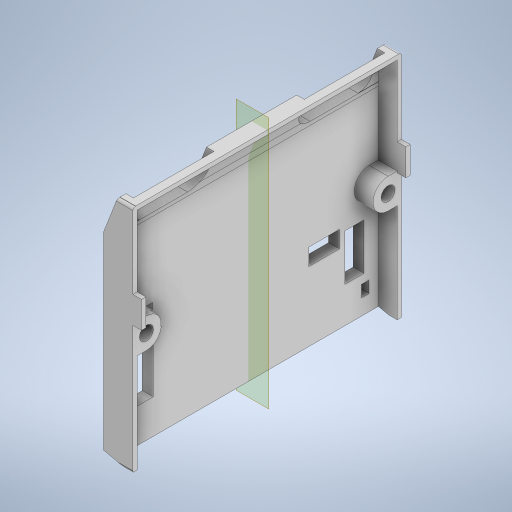
# Autodesk Inventor part: pokrywa
Saved by Autodesk Inventor 2023.5 (Build 275446000, 446)
## iProperties
Created: 2025-04-01
Part Number: pokrywa
Material: Ogólny
Document SubType Name: Modeling
Designer: kamil
Density: 1 g/cm^3
Appearance: Domyślna
Author: kamil
Autodesk Inventor part; units mm, degrees
ref_plane "YZ Plane" through (0, 0, 0) normal (1, 0, 0) x (0, 1, 0)
ref_plane "XZ Plane" through (0, 0, 0) normal (0, 1, 0) x (-1, 0, 0)
ref_plane "XY Plane" through (0, 0, 0) normal (0, 0, 1) x (1, 0, 0)
sketch "Szkic1" plane through (0, 0, 0) normal (1, 0, 0) x (0, 1, 0)
  line L0 (10.7442, -21.3655) -> (23.7442, -21.3655)
  line L1 (23.7442, -21.3655) -> (23.8098, -21.3634)
  arc A0 (23.8098, -21.3634) -> (24.2442, -20.8655) centre (23.7464, -20.8696) ccw
  line L2 (24.2442, -20.8655) -> (24.2442, 28.1345)
  line L3 (24.2442, 28.1345) -> (24.2421, 28.2)
  arc A1 (24.2421, 28.2) -> (23.7442, 28.6345) centre (23.7483, 28.1367) ccw
  line L4 (23.7442, 28.6345) -> (10.7442, 28.6345)
  line L5 (10.7442, 28.6345) -> (10.6787, 28.6324)
  line L6 (3.7484, 28.6345) -> (-18.1981, 28.6345)
  line L7 (-18.1981, 28.6345) -> (-18.2637, 28.6326)
  arc A2 (-18.2637, 28.6326) -> (-18.6981, 28.1345) centre (-18.2006, 28.139) ccw
  line L8 (-18.6981, 28.1345) -> (-18.6981, 27.1345)
  line L9 (-18.6981, 27.1345) -> (-18.6962, 27.0689)
  arc A3 (-18.6962, 27.0689) -> (-18.1981, 26.6345) centre (-18.2025, 27.1322) ccw
  line L10 (-18.1981, 26.6345) -> (-15.6162, 26.6345)
  line L11 (-15.6162, 26.6345) -> (-15.6162, 15.9345)
  line L12 (-15.6162, 15.9345) -> (-18.2023, 15.9345)
  line L13 (-18.2023, 15.9345) -> (-18.2679, 15.9326)
  arc A4 (-18.2679, 15.9326) -> (-18.7023, 15.4345) centre (-18.2048, 15.439) ccw
  line L14 (-18.7023, 15.4345) -> (-18.7023, -3.8655)
  line L15 (-18.7023, -3.8655) -> (-18.7004, -3.9311)
  arc A5 (-18.7004, -3.9311) -> (-18.2023, -4.3655) centre (-18.2067, -3.8678) ccw
  line L16 (-18.2023, -4.3655) -> (-15.6162, -4.3655)
  line L17 (-15.6162, -4.3655) -> (-15.6162, -15.0655)
  line L18 (-15.6162, -15.0655) -> (-18.2023, -15.0655)
  line L19 (-18.2023, -15.0655) -> (-18.2679, -15.0674)
  arc A6 (-18.2679, -15.0674) -> (-18.7023, -15.5655) centre (-18.2048, -15.561) ccw
  line L20 (-18.7023, -15.5655) -> (-18.7023, -20.8655)
  line L21 (-18.7023, -20.8655) -> (-18.7004, -20.9311)
  arc A7 (-18.7004, -20.9311) -> (-18.2023, -21.3655) centre (-18.2067, -20.8678) ccw
  line L22 (-18.2023, -21.3655) -> (3.7442, -21.3655)
  line L23 (3.7442, -21.3655) -> (3.8621, -21.3632)
  circle A8 centre (2.7442, 26.1345) radius 1.3
  circle A9 centre (2.7442, -18.8655) radius 1.3
  line L24 (10.7442, 28.6345) -> (3.7484, 28.6345)
  line L25 (3.7442, -21.3655) -> (10.7442, -21.3655)
  point P0 (0, 0)
  constraints: 52 end point, 16 point on circle, 10 centre point, 10 horizontal, 6 vertical, 1 parallel, 65 other
extrude "Wyciągnięcie proste1" add sketch "Szkic1" along normal blind 4
sketch "Szkic2" plane through (4, 0, 0) normal (1, 0, 0) x (0, 0, -1)
  line L0 (31.8312, -18.461) -> (-38.8363, -18.461)
  line L1 (21.3655, 23.7442) -> (21.3634, 23.8098) projected
  arc A0 (21.3634, 23.8098) -> (20.8655, 24.2442) centre (20.8696, 23.7464) ccw projected
  line L2 (20.8655, 24.2442) -> (-28.1345, 24.2442) projected
  line L3 (-28.1345, 24.2442) -> (-28.2, 24.2421) projected
  arc A1 (-28.2, 24.2421) -> (-28.6345, 23.7442) centre (-28.1367, 23.7483) ccw projected
  line L4 (-28.6345, 23.7442) -> (-28.6345, -18.1981) projected
  line L5 (-28.6345, -18.1981) -> (-28.6326, -18.2637) projected
  arc A2 (-28.6326, -18.2637) -> (-28.1345, -18.6981) centre (-28.139, -18.2006) ccw projected
  line L6 (-28.1345, -18.6981) -> (-27.1345, -18.6981) projected
  line L7 (-27.1345, -18.6981) -> (-27.0689, -18.6962) projected
  arc A3 (-27.0689, -18.6962) -> (-26.6345, -18.1981) centre (-27.1322, -18.2025) ccw projected
  line L8 (-26.6345, -18.1981) -> (-26.6345, -15.6162) projected
  line L9 (-26.6345, -15.6162) -> (-15.9345, -15.6162) projected
  line L10 (-15.9345, -15.6162) -> (-15.9345, -18.2023) projected
  line L11 (-15.9345, -18.2023) -> (-15.9326, -18.2679) projected
  arc A4 (-15.9326, -18.2679) -> (-15.4345, -18.7023) centre (-15.439, -18.2048) ccw projected
  line L12 (-15.4345, -18.7023) -> (3.8655, -18.7023) projected
  line L13 (3.8655, -18.7023) -> (3.9311, -18.7004) projected
  arc A5 (3.9311, -18.7004) -> (4.3655, -18.2023) centre (3.8678, -18.2067) ccw projected
  line L14 (4.3655, -18.2023) -> (4.3655, -15.6162) projected
  line L15 (4.3655, -15.6162) -> (15.0655, -15.6162) projected
  line L16 (15.0655, -15.6162) -> (15.0655, -18.2023) projected
  line L17 (15.0655, -18.2023) -> (15.0674, -18.2679) projected
  arc A6 (15.0674, -18.2679) -> (15.5655, -18.7023) centre (15.561, -18.2048) ccw projected
  line L18 (15.5655, -18.7023) -> (20.8655, -18.7023) projected
  line L19 (20.8655, -18.7023) -> (20.9311, -18.7004) projected
  arc A7 (20.9311, -18.7004) -> (21.3655, -18.2023) centre (20.8678, -18.2067) ccw projected
  line L20 (21.3655, -18.2023) -> (21.3655, 23.7442) projected
  circle A8 centre (-26.1345, 2.7442) radius 1.3 projected
  circle A9 centre (18.8655, 2.7442) radius 1.3 projected
  line L21 (20.8655, 24.2442) -> (-28.1345, 24.2442) projected
  point P0 (0, 0)
  point P1 (-26.7069, -18.461)
  point P2 (-15.8655, -18.461)
  point P3 (4.2957, -18.461)
  point P4 (15.1345, -18.461)
  point P5 (21.2957, -18.461)
  point P6 (-28.563, -18.461)
  constraints: 2 end point, 1 parallel
extrude "Wyciągnięcie proste2" add sketch "Szkic2" against normal up to surface (4 mm away) contours L0 A5 L14 L15 L16 L17 A6 | L0 A3 L8 L9 L10 L11 A4
extrude "Wyciągnięcie proste3" cut sketch "Szkic2" against normal through all contours A7 L19 L18 A6 L0 | A5 L13 L12 A4 L0 | A3 L7 L6 A2 L0
sketch "Szkic4" plane through (4, 0, 0) normal (1, 0, 0) x (0, 0, -1)
  circle A0 centre (18.8655, 2.7442) radius 1.3 projected
  circle A1 centre (-26.1345, 2.7442) radius 1.3 projected
  line L0 (-28.563, -18.461) -> (21.2957, -18.461) projected
  arc A2 (21.2957, -18.461) -> (21.3655, -18.2023) centre (20.8678, -18.2067) ccw projected
  line L1 (21.3655, -18.2023) -> (21.3655, 23.7442) projected
  line L2 (21.3655, 23.7442) -> (21.3634, 23.8098) projected
  arc A3 (21.3634, 23.8098) -> (20.8655, 24.2442) centre (20.8696, 23.7464) ccw projected
  line L3 (20.8655, 24.2442) -> (-28.1345, 24.2442) projected
  line L4 (-28.1345, 24.2442) -> (-28.2, 24.2421) projected
  arc A4 (-28.2, 24.2421) -> (-28.6345, 23.7442) centre (-28.1367, 23.7483) ccw projected
  line L5 (-28.6345, 23.7442) -> (-28.6345, -18.1981) projected
  line L6 (-28.6345, -18.1981) -> (-28.6326, -18.2637) projected
  arc A5 (-28.6326, -18.2637) -> (-28.563, -18.461) centre (-28.139, -18.2006) ccw projected
  line L7 (20.5655, 23.4442) -> (20.5655, -17.661)
  line L8 (20.5655, -17.661) -> (-27.8345, -17.661)
  line L9 (-27.8345, -17.661) -> (-27.8345, 23.4442)
  line L10 (-27.8345, 23.4442) -> (20.5655, 23.4442)
  circle A6 centre (18.8655, 2.7442) radius 2.8
  circle A7 centre (-26.1345, 2.7442) radius 2.8
  line L11 (18.8655, -0.0558) -> (20.5655, -0.0558)
  line L12 (20.5655, 5.5442) -> (18.8655, 5.5442)
  line L13 (-26.1345, -0.0558) -> (-27.8345, -0.0558)
  line L14 (-26.1345, 5.5442) -> (-27.8345, 5.5442)
  point P0 (0, 0)
  dimension "d8" = 0.8
  dimension "d9" = 1.5
  dimension "d10" = 1.5
  constraints: 16 end point, 4 perpendicular, 4 point on circle, 4 point on line, 4 tangent, 2 centre point, 3 other
  measures "d8" distance between parallel lines of L1 L7
  measures "d9" radial gap between concentric circles of A0 A6
  measures "d10" radial gap between concentric circles of A1 A7
extrude "Wyciągnięcie proste5" cut sketch "Szkic4" against normal blind 2 contours L7 L8 L9 L13 A7 L14 L10 L12 A6 L11
sketch "Szkic5" plane through (4, 0, 0) normal (1, 0, 0) x (0, 0, -1)
  line L0 (18.8655, -0.0558) -> (20.5655, -0.0558) projected
  line L1 (20.5655, -0.0558) -> (20.5655, -17.661) projected
  line L2 (20.5655, -17.661) -> (-27.8345, -17.661) projected
  line L3 (-27.8345, -17.661) -> (-27.8345, -0.0558) projected
  line L4 (-27.8345, -0.0558) -> (-26.1345, -0.0558) projected
  arc A0 (-26.1345, -0.0558) -> (-26.1345, 5.5442) centre (-26.1345, 2.7442) ccw projected
  line L5 (-26.1345, 5.5442) -> (-27.8345, 5.5442) projected
  line L6 (-27.8345, 5.5442) -> (-27.8345, 23.4442) projected
  line L7 (-27.8345, 23.4442) -> (20.5655, 23.4442) projected
  line L8 (20.5655, 23.4442) -> (20.5655, 5.5442) projected
  line L9 (20.5655, 5.5442) -> (18.8655, 5.5442) projected
  arc A1 (18.8655, 5.5442) -> (18.8655, -0.0558) centre (18.8655, 2.7442) ccw projected
  circle A2 centre (18.8655, 2.7442) radius 1.3 projected
  circle A3 centre (-26.1345, 2.7442) radius 1.3 projected
  line L10 (-28.563, -18.461) -> (21.2957, -18.461) projected
  arc A4 (21.2957, -18.461) -> (21.3655, -18.2023) centre (20.8678, -18.2067) ccw projected
  line L11 (21.3655, -18.2023) -> (21.3655, 23.7442) projected
  line L12 (21.3655, 23.7442) -> (21.3634, 23.8098) projected
  arc A5 (21.3634, 23.8098) -> (20.8655, 24.2442) centre (20.8696, 23.7464) ccw projected
  line L13 (20.8655, 24.2442) -> (-28.1345, 24.2442) projected
  line L14 (-28.1345, 24.2442) -> (-28.2, 24.2421) projected
  arc A6 (-28.2, 24.2421) -> (-28.6345, 23.7442) centre (-28.1367, 23.7483) ccw projected
  line L15 (-28.6345, 23.7442) -> (-28.6345, -18.1981) projected
  line L16 (-28.6345, -18.1981) -> (-28.6326, -18.2637) projected
  arc A7 (-28.6326, -18.2637) -> (-28.563, -18.461) centre (-28.139, -18.2006) ccw projected
  point P0 (0, 0)
extrude "Wyciągnięcie proste6" add sketch "Szkic5" along normal blind 1.5
sketch "Szkic9" plane through (0, 0, 0) normal (-1, 0, 0) x (0, 0, 1)
  line L0 (-21.2957, -18.461) -> (28.563, -18.461) projected
  arc A0 (28.563, -18.461) -> (28.6326, -18.2637) centre (28.139, -18.2006) ccw projected
  line L1 (28.6345, -18.1981) -> (28.6326, -18.2637) projected
  line L2 (28.6345, 23.7442) -> (28.6345, -18.1981) projected
  arc A1 (28.6345, 23.7442) -> (28.2, 24.2421) centre (28.1367, 23.7483) ccw projected
  line L3 (28.1345, 24.2442) -> (28.2, 24.2421) projected
  line L4 (-20.8655, 24.2442) -> (28.1345, 24.2442) projected
  arc A2 (-20.8655, 24.2442) -> (-21.3634, 23.8098) centre (-20.8696, 23.7464) ccw projected
  line L5 (-21.3655, 23.7442) -> (-21.3634, 23.8098) projected
  line L6 (-21.3655, -18.2023) -> (-21.3655, 23.7442) projected
  arc A3 (-21.3655, -18.2023) -> (-21.2957, -18.461) centre (-20.8678, -18.2067) ccw projected
  circle A4 centre (26.1345, 2.7442) radius 1.3 projected
  circle A5 centre (-18.8655, 2.7442) radius 1.3 projected
  line L7 (27.0345, 24.2442) -> (12.0345, 24.2442)
  line L8 (12.0345, 24.2442) -> (12.0345, 18.2442)
  line L9 (12.0345, 18.2442) -> (27.0345, 18.2442)
  line L10 (27.0345, 18.2442) -> (27.0345, 24.2442)
  line L11 (-19.7655, 24.2442) -> (-4.7655, 24.2442)
  line L12 (-4.7655, 24.2442) -> (-4.7655, 18.2442)
  line L13 (-4.7655, 18.2442) -> (-19.7655, 18.2442)
  line L14 (-19.7655, 18.2442) -> (-19.7655, 24.2442)
  line L15 (-20.8655, 24.2442) -> (28.1345, 24.2442) projected
  point P0 (0, 0)
  point P1 (-4.7655, 24.2442)
  point P2 (-19.7655, 24.2442)
  dimension "d20" = 15
  dimension "d21" = 15
  dimension "d22" = 1.6
  dimension "d23" = 1.6
  dimension "d24" = 6
  constraints: 16 end point, 4 parallel, 2 collinear, 2 horizontal, 2 perpendicular, 1 point on line
  measures "d20" distance between parallel lines of L8 L10
  measures "d21" distance between parallel lines of L14 L12
  measures "d22" distance between parallel lines of L10 L2
  measures "d23" distance between parallel lines of L6 L14
  measures "d24" distance between parallel lines of L7 L9
extrude "Wyciągnięcie proste9" cut sketch "Szkic9" against normal blind 4 contours L4 L12 L13 L14 | L10 L9 L8 L4
sketch "Szkic10" plane through (0, 18.2442, 12.0345) normal (0, 0, 1) x (1, 0, 0)
  line L0 (2, 5.2) -> (2, 0) projected
  line L1 (4, 5.2) -> (2, 5.2) projected
  line L2 (4, 5.2) -> (4, 6) projected
  line L3 (0, 6) -> (4, 6) projected
  line L4 (0, 0) -> (0, 6) projected
  line L5 (0, 0) -> (2, 0) projected
  line L6 (2, 5.2) -> (2, 0) projected
  line L7 (4, 5.2) -> (2, 5.2) projected
  line L8 (2, 0) -> (4, 5.2)
  point P0 (0, -18.2442)
  constraints: 2 end point
extrude "Wyciągnięcie proste10" add sketch "Szkic10" against normal up to surface (16.8 mm away) contours L1 L8 L0
sketch "Szkic11" plane through (0, -18.1981, 28.6345) normal (0, 0, 1) x (1, 0, 0)
  line L0 (2, 36.4423) -> (4, 41.6423) projected
  line L1 (-3.0884, 27.6697) -> (6.2618, 51.9802)
  line L2 (0, 42.4402) -> (0, 41.9423) projected
  line L3 (0, 41.9423) -> (5.5, 41.9423) projected
  line L4 (5.5, 42.4402) -> (5.5, 41.9423) projected
  line L5 (0, 42.4402) -> (5.5, 42.4402) projected
  line L6 (0, 41.9423) -> (0, 0) projected
  line L7 (0, 0) -> (5.5, 0) projected
  line L8 (5.5, 41.9423) -> (5.5, 0) projected
  line L9 (0, 41.9423) -> (5.5, 41.9423) projected
  line L10 (-3.0884, 27.6697) -> (-8.821, 53.9859)
  line L11 (-8.821, 53.9859) -> (6.2618, 51.9802)
  point P0 (0, 18.1981)
  dimension "d29" = 1.6
  constraints: 6 end point, 1 parallel
  measures "d29" distance between parallel lines of L1 L0
extrude "Wyciągnięcie proste11" cut sketch "Szkic11" along normal blind 10 and the other way blind 100 contours L10 L11 L1 L5 L2 L6 | L6 L3 L1 | L3 L2 L5 L1
sketch "Szkic12" plane through (2, 5.5442, -20.5655) normal (0, 0, 1) x (1, 0, 0)
  line L0 (0, 17.1571) -> (-1.7143, 12.7) projected
  line L1 (0.5934, 18.7) -> (0.2857, 17.9) projected
  line L2 (0.2857, 17.9) -> (0, 17.1571) projected
  line L3 (-0.7809, 12.341) -> (0.9333, 16.7981)
  line L4 (0.9333, 16.7981) -> (1.2191, 17.541)
  line L5 (1.2191, 17.541) -> (1.5268, 18.341)
  line L6 (0.2857, 17.9) -> (0, 17.1571) projected
  line L7 (0, 17.1571) -> (0, 0) projected
  line L8 (3.5, 0) -> (0, 0) projected
  line L9 (3.5, 17.9) -> (3.5, 0) projected
  line L10 (3.5, 17.9) -> (0.2857, 17.9) projected
  point P0 (-2, -5.5442)
  point P1 (1.3572, 17.9)
  point P2 (0, 14.3714)
  dimension "d34" = 1
  constraints: 6 end point, 2 other
  measures "d34" distance between parallel lines of L2 L4
extrude "Wyciągnięcie proste12" add sketch "Szkic12" along normal up to surface (0.8 mm away) contours L10 L5 L4 L3 L7 L2
ref_plane "Płaszczyzna konstrukcyjna1" through (5.5, -18.2023, 3.6345) normal (0, 0, -1) x (-1, 0, 0)
mirror "Odbij1" about plane through (5.5, -18.2023, 3.6345) normal (0, 0, -1) of "Wyciągnięcie proste12"
sketch "Szkic13" plane through (0, -18.1981, 28.6345) normal (0, 0, 1) x (1, 0, 0)
  line L0 (9.4474, -1.511) -> (-6.0785, 1.9749)
  line L1 (5.5, -0.2629) -> (0, -0.2629) projected
  line L2 (0, -0.2629) -> (0.1866, 0.5682)
  line L3 (0, -0.2629) -> (5.5, -0.2629) projected
  line L4 (5.5, -0.0656) -> (5.5, -0.2629) projected
  line L5 (0, -0.0656) -> (5.5, -0.0656) projected
  line L6 (0, -0.0656) -> (0, -0.2629) projected
  line L7 (2.4011, 41.9423) -> (0, 35.6994) projected
  line L8 (0, 35.6994) -> (0, 0) projected
  line L9 (0, 0) -> (5.5, 0) projected
  line L10 (5.5, 41.9423) -> (5.5, 0) projected
  line L11 (2.4011, 41.9423) -> (5.5, 41.9423) projected
  line L12 (0, 0) -> (5.5, 0) projected
  line L13 (0, 0) -> (0, -0.0656) projected
  line L14 (0, -0.0656) -> (5.5, -0.0656) projected
  line L15 (5.5, 0) -> (5.5, -0.0656) projected
  line L16 (0, 0) -> (5.5, 0) projected
  point P0 (0, 18.1981)
  point P1 (0, 0.6101)
  point P2 (3.8884, -0.2629)
  constraints: 4 end point, 1 perpendicular, 1 point on line
extrude "Wyciągnięcie proste13" cut sketch "Szkic13" against normal through all contours L1 L2 L5 L0 | L5 L2 L9 L0 | L6 L5 L2 | L9 L2 L0 | L5 L13 L9 L2 | L2 L9 L8 L0
sketch "Szkic14" plane through (0, 0, 0) normal (-1, 0, 0) x (0, 0, 1)
  line L0 (-15.0995, -3.2358) -> (-17.1315, -3.2358) projected
  line L1 (-17.1315, -10.8558) -> (-15.0995, -10.8558) projected
  line L2 (-17.3855, -8.5698) -> (-17.3855, -10.6018) projected
  line L3 (-14.8455, -5.5218) -> (-14.8455, -3.4898) projected
  line L4 (24.4295, -11.1458) -> (21.8895, -11.1458)
  line L5 (21.8895, -11.1458) -> (21.8895, -0.9858)
  line L6 (21.8895, -0.9858) -> (24.4295, -0.9858)
  line L7 (24.4295, -0.9858) -> (24.4295, -11.1458)
  line L8 (-17.3855, -10.8558) -> (-14.8455, -10.8558)
  line L9 (-14.8455, -10.8558) -> (-14.8455, -3.2358)
  line L10 (-14.8455, -3.2358) -> (-17.3855, -3.2358)
  line L11 (-17.3855, -3.2358) -> (-17.3855, -10.8558)
  line L12 (-14.3455, -2.7358) -> (-14.3455, -11.3558)
  line L13 (-14.3455, -11.3558) -> (-17.8855, -11.3558)
  line L14 (-17.8855, -11.3558) -> (-17.8855, -2.7358)
  line L15 (-17.8855, -2.7358) -> (-14.3455, -2.7358)
  line L16 (21.3895, -0.4858) -> (21.3895, -11.6458)
  line L17 (21.3895, -11.6458) -> (24.9295, -11.6458)
  line L18 (24.9295, -11.6458) -> (24.9295, -0.4858)
  line L19 (24.9295, -0.4858) -> (21.3895, -0.4858)
  point P0 (0, 0)
  dimension "d40" = 0.5
  dimension "d41" = 0.5
  constraints: 32 end point, 8 parallel, 4 perpendicular, 2 horizontal, 8 other
  measures "d40" distance between parallel lines of L9 L12
  measures "d41" distance between parallel lines of L5 L16
extrude "Wyciągnięcie proste14" cut sketch "Szkic14" against normal through all contours L10 L9 L3 L8 L1 L11 L2 L0 | L4 L5 L6 L7 | L12 L13 L14 L15 | L19 L18 L17 L16
sketch "Szkic15" plane through (0, 0, 0) normal (-1, 0, 0) x (0, 0, 1)
  line L0 (23.2345, 2.6442) -> (21.6645, 2.6442)
  line L1 (21.6645, 2.6442) -> (21.6645, 3.4442)
  line L2 (21.6645, 3.4442) -> (23.2345, 3.4442)
  line L3 (23.2345, 3.4442) -> (23.2345, 2.6442)
  line L4 (23.4345, 3.6442) -> (21.4645, 3.6442)
  line L5 (21.4645, 3.6442) -> (21.4645, 2.4442)
  line L6 (21.4645, 2.4442) -> (23.4345, 2.4442)
  line L7 (23.4345, 2.4442) -> (23.4345, 3.6442)
  point P0 (0, 0)
  dimension "d44" = 0.2
  constraints: 16 end point, 4 parallel, 2 perpendicular, 1 horizontal, 5 other
  measures "d44" distance between parallel lines of L2 L4
extrude "Wyciągnięcie proste15" cut sketch "Szkic15" against normal through all contours L0 L1 L2 L3 | L7 L6 L5 L4
sketch "Szkic16" plane through (0, 0, 0) normal (-1, 0, 0) x (0, 0, 1)
  line L0 (-18.5155, -13.2058) -> (-17.7155, -13.2058)
  line L1 (-17.7155, -13.2058) -> (-17.7155, -14.7758)
  line L2 (-17.7155, -14.7758) -> (-18.5155, -14.7758)
  line L3 (-18.5155, -14.7758) -> (-18.5155, -13.2058)
  line L4 (-17.4155, -15.0758) -> (-17.4155, -12.9058)
  line L5 (-17.4155, -12.9058) -> (-18.8155, -12.9058)
  line L6 (-18.8155, -12.9058) -> (-18.8155, -15.0758)
  line L7 (-18.8155, -15.0758) -> (-17.4155, -15.0758)
  point P0 (0, 0)
  dimension "d47" = 0.3
  constraints: 16 end point, 4 parallel, 2 perpendicular, 1 horizontal, 5 other
  measures "d47" distance between parallel lines of L1 L4
extrude "Wyciągnięcie proste16" cut sketch "Szkic16" against normal through all contours L0 L1 L2 L3 | L7 L6 L5 L4
sketch "Szkic17" plane through (5.5, 0, 0) normal (1, 0, 0) x (0, 0, -1)
  circle A0 centre (-26.1345, 2.7442) radius 1.3 projected
  circle A1 centre (18.8655, 2.7442) radius 1.3 projected
  line L0 (-23.3506, 2.4442) -> (-23.4345, 2.4442) projected
  line L1 (-23.4345, 2.4442) -> (-23.4345, 3.4859) projected
  arc A2 (-23.4345, 3.4859) -> (-26.1345, 5.5442) centre (-26.1345, 2.7442) ccw projected
  line L2 (-26.1345, 5.5442) -> (-27.8345, 5.5442) projected
  line L3 (-27.8345, 5.5442) -> (-27.8345, 23.4442) projected
  line L4 (-27.8345, 23.4442) -> (20.5655, 23.4442) projected
  line L5 (20.5655, 23.4442) -> (20.5655, 5.5442) projected
  line L6 (20.5655, 5.5442) -> (18.8655, 5.5442) projected
  arc A3 (18.8655, 5.5442) -> (18.8655, -0.0558) centre (18.8655, 2.7442) ccw projected
  line L7 (18.8655, -0.0558) -> (20.5655, -0.0558) projected
  line L8 (20.5655, -0.0558) -> (20.5655, -17.661) projected
  line L9 (20.5655, -17.661) -> (-27.8345, -17.661) projected
  line L10 (-27.8345, -17.661) -> (-27.8345, -0.0558) projected
  line L11 (-27.8345, -0.0558) -> (-26.1345, -0.0558) projected
  arc A4 (-26.1345, -0.0558) -> (-23.3506, 2.4442) centre (-26.1345, 2.7442) ccw projected
  arc A5 (21.2957, -18.461) -> (21.3655, -18.2023) centre (20.8678, -18.2067) ccw projected
  line L12 (21.3655, -18.2023) -> (21.3655, 23.7442) projected
  line L13 (21.3655, 23.7442) -> (21.3634, 23.8098) projected
  arc A6 (21.3634, 23.8098) -> (20.8655, 24.2442) centre (20.8696, 23.7464) ccw projected
  line L14 (20.8655, 24.2442) -> (-28.1345, 24.2442) projected
  line L15 (-28.1345, 24.2442) -> (-28.2, 24.2421) projected
  arc A7 (-28.2, 24.2421) -> (-28.6345, 23.7442) centre (-28.1367, 23.7483) ccw projected
  line L16 (-28.6345, 23.7442) -> (-28.6345, -18.1981) projected
  line L17 (-28.6345, -18.1981) -> (-28.6326, -18.2637) projected
  arc A8 (-28.6326, -18.2637) -> (-28.563, -18.461) centre (-28.139, -18.2006) ccw projected
  line L18 (-28.563, -18.461) -> (21.2957, -18.461) projected
  line L19 (-27.8345, -17.661) -> (-27.8345, -0.0558) projected
  line L20 (-27.8345, -17.661) -> (20.5655, -17.661)
  line L21 (20.5655, -17.661) -> (20.5655, -23.8165)
  line L22 (20.5655, -23.8165) -> (-27.8345, -23.8165)
  line L23 (-27.8345, -23.8165) -> (-27.8345, -17.661)
  point P0 (0, 0)
  constraints: 8 end point, 2 parallel, 1 horizontal, 1 perpendicular
extrude "Wyciągnięcie proste17" cut sketch "Szkic17" against normal up to surface (3.5 mm away) contours L9 L21 L18 L23 | L18 L21 L22 L23
sketch "Szkic18" plane through (0, 0, 0) normal (-1, 0, 0) x (0, 0, 1)
  line L0 (-13.0005, -4.5718) -> (-13.0005, -2.5398) projected
  line L1 (-12.7465, -2.2858) -> (-10.7145, -2.2858) projected
  line L2 (-7.9205, -2.5398) -> (-7.9205, -4.5718) projected
  line L3 (-8.1745, -4.8258) -> (-10.2065, -4.8258) projected
  line L4 (-13.0005, -2.2858) -> (-7.9205, -2.2858)
  line L5 (-7.9205, -2.2858) -> (-7.9205, -4.8258)
  line L6 (-7.9205, -4.8258) -> (-13.0005, -4.8258)
  line L7 (-13.0005, -4.8258) -> (-13.0005, -2.2858)
  line L8 (-7.6205, -1.9858) -> (-13.3005, -1.9858)
  line L9 (-13.3005, -1.9858) -> (-13.3005, -5.1258)
  line L10 (-13.3005, -5.1258) -> (-7.6205, -5.1258)
  line L11 (-7.6205, -5.1258) -> (-7.6205, -1.9858)
  point P0 (0, 0)
  dimension "d52" = 0.3
  constraints: 16 end point, 4 parallel, 2 perpendicular, 1 horizontal, 3 other
  measures "d52" distance between parallel lines of L4 L8
extrude "Wyciągnięcie proste18" cut sketch "Szkic18" against normal through all contours L0 L7 L4 L1 L5 L2 L6 L3 | L11 L10 L9 L8
sketch "Szkic19" plane through (5.5, 0, 0) normal (1, 0, 0) x (0, 0, -1)
  line L0 (-28.1345, 10.2442) -> (-20.8845, 10.2442) projected
  line L1 (-20.8845, 5.2442) -> (-27.1345, 5.2442) projected
  line L2 (20.5655, -0.0558) -> (20.5655, -18.461) projected
  line L3 (-28.563, -18.461) -> (-27.8345, -18.461) projected
  arc A0 (21.2957, -18.461) -> (21.3655, -18.2023) centre (20.8678, -18.2067) ccw projected
  line L4 (21.3655, -18.2023) -> (21.3655, 23.7442) projected
  line L5 (21.3655, 23.7442) -> (21.3634, 23.8098) projected
  arc A1 (21.3634, 23.8098) -> (20.8655, 24.2442) centre (20.8696, 23.7464) ccw projected
  line L6 (20.8655, 24.2442) -> (-28.1345, 24.2442) projected
  line L7 (-28.1345, 24.2442) -> (-28.2, 24.2421) projected
  arc A2 (-28.2, 24.2421) -> (-28.6345, 23.7442) centre (-28.1367, 23.7483) ccw projected
  line L8 (-28.6345, 23.7442) -> (-28.6345, -18.1981) projected
  line L9 (-28.6345, -18.1981) -> (-28.6326, -18.2637) projected
  arc A3 (-28.6326, -18.2637) -> (-28.563, -18.461) centre (-28.139, -18.2006) ccw projected
  line L10 (20.5655, -18.461) -> (21.2957, -18.461) projected
  line L11 (-27.8345, -18.461) -> (-27.8345, -0.0558) projected
  line L12 (-27.8345, -0.0558) -> (-26.1345, -0.0558) projected
  arc A4 (-26.1345, -0.0558) -> (-23.3506, 2.4442) centre (-26.1345, 2.7442) ccw projected
  line L13 (-23.3506, 2.4442) -> (-23.4345, 2.4442) projected
  line L14 (-23.4345, 2.4442) -> (-23.4345, 3.4859) projected
  arc A5 (-23.4345, 3.4859) -> (-26.1345, 5.5442) centre (-26.1345, 2.7442) ccw projected
  line L15 (-26.1345, 5.5442) -> (-27.8345, 5.5442) projected
  line L16 (-27.8345, 5.5442) -> (-27.8345, 23.4442) projected
  line L17 (-27.8345, 23.4442) -> (20.5655, 23.4442) projected
  line L18 (20.5655, 23.4442) -> (20.5655, 5.5442) projected
  line L19 (20.5655, 5.5442) -> (18.8655, 5.5442) projected
  arc A6 (18.8655, 5.5442) -> (18.8655, -0.0558) centre (18.8655, 2.7442) ccw projected
  line L20 (18.8655, -0.0558) -> (20.5655, -0.0558) projected
  circle A7 centre (18.8655, 2.7442) radius 1.3 projected
  circle A8 centre (-26.1345, 2.7442) radius 1.3 projected
  line L21 (19.8655, 5.2442) -> (13.6155, 5.2442) projected
  line L22 (13.6155, 10.2442) -> (20.8655, 10.2442) projected
  line L23 (-28.1345, 10.2442) -> (-28.6345, 10.2442)
  line L24 (-27.1345, 5.2442) -> (-28.6345, 5.2442)
  line L25 (-26.1345, 5.5442) -> (-27.8345, 5.5442) projected
  line L26 (-27.8345, 5.5442) -> (-27.8345, 5.2442)
  line L27 (20.8655, 10.2442) -> (21.3655, 10.2442)
  line L28 (21.3655, -17.588) -> (21.3655, 17.5013) projected
  line L29 (19.8655, 5.2442) -> (21.3655, 5.2442)
  line L30 (20.5655, 5.5442) -> (20.5655, 5.2442)
  point P0 (0, 0)
  point P1 (-27.8345, 10.2442)
  point P2 (20.5655, 10.2442)
  constraints: 12 end point, 6 point on line, 5 perpendicular, 1 horizontal
extrude "Wyciągnięcie proste19" add sketch "Szkic19" along normal blind 1.6 contours L0 L16 L26 L24 L8 L23 | L22 L27 L4 L29 L30 L18
fillet "Zaokrąglenie2" radius 4 1 edges at (2, 18.2442, 3.6345)
fillet "Zaokrąglenie3" radius 3 4 edges at (1.1776, 18.2442, 12.0345) (1.1429, 18.2442, -19.7655) (1.1776, 18.2442, -4.7655) (1.1429, 18.2442, 27.0345)
